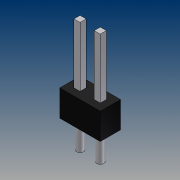
# Autodesk Inventor part: Jumper 2 Pin
Saved by Autodesk Inventor 2012 (Build 160160000, 160)
## iProperties
Company: Team 801
Created: 2007-11-01
Part Number: Jumper 2 Pin
Document SubType Name: Modeling
Designer: Jeffrey M
Manufacturer: Standard
Standards Organization: Custom
Mass: 0.0555648 g
Surface Area: 1.4096 cm^2
Volume: 0.0555648 cm^3
Density: 1 g/cm^3
Catalog Web Link: www.team801.org
Material: Default
PartAngTol0: 0.50 deg
PartAngTol1: 0.50 deg
PartAngTol2: 0.50 deg
PartLinTol0: 0.01 in
PartLinTol1: 0.01 in
PartLinTol2: 0.01 in
PartLinTol3: 0.005 in
PartAngTol3: 0deg30'
Author: Jeffrey M
Autodesk Inventor part; units mm, degrees
ref_plane "YZ Plane (RIGHT)" through (0, 0, 0) normal (1, 0, 0) x (0, 1, 0)
ref_plane "XZ Plane (TOP)" through (0, 0, 0) normal (0, 1, 0) x (-1, 0, 0)
ref_plane "XY Plane (FRONT)" through (0, 0, 0) normal (0, 0, 1) x (1, 0, 0)
sketch "Sketch2" plane through (0, 0, 0) normal (0, 0, 1) x (1, 0, 0)
  line L0 (-1.778, 0) -> (1.778, 0) construction
  line L1 (0, 3.9624) -> (0, -0.6604) construction
  line L2 (-1.27, 3.302) -> (1.27, 3.302)
  line L3 (1.27, 3.302) -> (1.27, 0)
  line L4 (1.27, 0) -> (-1.27, 0)
  line L5 (-1.27, 0) -> (-1.27, 3.302)
  point P0 (0, 0)
  dimension "d0" = 2.54
  dimension "d1" = 3.302
  constraints: 8 end point, 2 parallel, 1 horizontal, 1 perpendicular, 1 point on line, 1 other
  measures "d0" distance of L2.start L2.end
  measures "d1" distance of L4.end L2.start
extrude "Extrusion1" add sketch "Sketch2" along normal mid plane 2.54
sketch "Sketch3" plane through (-1.27, 0, 1.27) normal (0, -1, 0) x (1, 0, 0)
  circle A0 centre (1.27, -1.27) radius 0.4445
  line L0 (1.27, 0.508) -> (1.27, -3.048) construction
  line L1 (-0.508, -1.27) -> (3.048, -1.27) construction
  line L2 (0.889, -0.889) -> (1.651, -0.889)
  line L3 (1.651, -0.889) -> (1.651, -1.651)
  line L4 (1.651, -1.651) -> (0.889, -1.651)
  line L5 (0.889, -1.651) -> (0.889, -0.889)
  dimension "d4" = 0.762
  dimension "d5" = 0.889
  constraints: 8 end point, 2 parallel, 2 perpendicular, 1 centre point, 1 coincident, 1 horizontal, 2 other
  measures "d4" distance of L2.start L2.end
  measures "d5" diameter of A0
extrude "Extrusion2" add sketch "Sketch3" against normal blind 10.795 contours L3 A0 L4 L5 L2 | A0 L2 L3 | L3 L4 A0 | A0 L5 L2 | L4 L5 A0
extrude "Extrusion3" add sketch "Sketch3" along normal blind 3.429 contours A0 L3 | L3 A0 L4 L5 L2 | L2 A0 | A0 L4 | L5 A0
pattern_linear "Rectangular Pattern1" count 2 spacing 2.54 along (1, 0, 0) of "Extrusion1", "Extrusion2", "Extrusion3"
body "Solid1"
